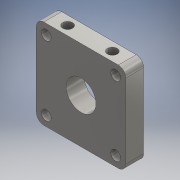
# Autodesk Inventor part: Bearing_Block
Saved by Autodesk Inventor 2016 (Build 200138000, 138)
## iProperties
Created: 2016-04-11
Part Number: Bearing_Block
Material: Steel, Mild
Document SubType Name: Modeling
Designer: agmle
Density: 7.85 g/cm^3
Appearance: Semi-Polished
Author: agmle
Autodesk Inventor part; units mm, degrees
ref_plane "YZ Plane" through (0, 0, 0) normal (1, 0, 0) x (0, 1, 0)
ref_plane "XZ Plane" through (0, 0, 0) normal (0, 1, 0) x (-1, 0, 0)
ref_plane "XY Plane" through (0, 0, 0) normal (0, 0, 1) x (1, 0, 0)
sketch "Sketch1" plane through (0, 0, 0) normal (0, 1, 0) x (-1, 0, 0)
  line L0 (16.6369, 20.0223) -> (-15.1131, 20.0223)
  line L1 (-18.2881, 16.8473) -> (-18.2881, -14.9027)
  line L2 (-15.1131, -18.0777) -> (16.6369, -18.0777)
  line L3 (19.8119, -14.9027) -> (19.8119, 16.8473)
  arc A0 (19.8119, 16.8473) -> (16.6369, 20.0223) centre (16.6369, 16.8473) ccw
  arc A1 (-18.2881, -14.9027) -> (-15.1131, -18.0777) centre (-15.1131, -14.9027) ccw
  arc A2 (16.6369, -18.0777) -> (19.8119, -14.9027) centre (16.6369, -14.9027) ccw
  arc A3 (-15.1131, 20.0223) -> (-18.2881, 16.8473) centre (-15.1131, 16.8473) ccw
  point P0 (0, 0)
  dimension "d0" = 38.1
  dimension "d1" = 3.175
  constraints: 8 end point, 8 point on circle, 8 tangent, 4 centre point, 3 equal radius, 2 parallel, 2 perpendicular, 1 horizontal
  measures "d0" distance between parallel lines of L2 L0
  measures "d1" radius of A0
extrude "Extrusion1" add sketch "Sketch1" along normal blind 7.62
sketch "Sketch2" plane through (0, 7.62, 0) normal (0, 1, 0) x (1, 0, 0)
  line L0 (-19.8119, 14.9027) -> (-19.8119, -16.8473) projected
  line L1 (-16.6369, -20.0223) -> (15.1131, -20.0223) projected
  line L2 (15.1131, 18.0777) -> (-16.6369, 18.0777) projected
  line L3 (18.2881, -16.8473) -> (18.2881, 14.9027) projected
  point P0 (0, 0)
  point P1 (-15.5619, -15.7723)
  point P2 (-15.5619, 13.8277)
  point P3 (14.0381, 13.8277)
  point P4 (14.0381, -15.7723)
  dimension "d4" = 4.25
  dimension "d5" = 4.25
  dimension "d6" = 4.25
  dimension "d7" = 4.25
  dimension "d8" = 4.25
  dimension "d9" = 4.25
  dimension "d10" = 4.25
  dimension "d11" = 4.25
  measures "d4" distance from line of L0 point (-15.562, -15.772)
  measures "d5" distance from line of L1 point (-15.562, -15.772)
  measures "d6" distance from line of L0 point (-15.562, 13.828)
  measures "d7" distance from line of L2 point (-15.562, 13.828)
  measures "d8" distance from line of L2 point (14.038, 13.828)
  measures "d9" distance from line of L3 point (14.038, 13.828)
  measures "d10" distance from line of L3 point (14.038, -15.772)
  measures "d11" distance from line of L1 point (14.038, -15.772)
hole "Hole1" at (-15.5619, 7.62, 15.7723) at (-15.5619, 7.62, -13.8277) at (14.0381, 7.62, -13.8277) at (14.0381, 7.62, 15.7723) direction (0, -1, 0) diameter 4.2 end through all
sketch "Sketch3" plane through (0, 7.62, 0) normal (0, 1, 0) x (1, 0, 0)
  line L0 (-19.8119, 14.9027) -> (-19.8119, -16.8473) construction
  line L1 (-19.8119, -0.9723) -> (18.2881, -0.9723) construction
  line L2 (18.2881, -16.8473) -> (18.2881, 14.9027) construction
  point P0 (0, 0)
  point P1 (-0.7619, -0.9723)
  point P2 (-0.7619, -0.9723)
  constraints: 3 midpoint, 2 end point, 1 coincident
hole "Hole2" at (-0.7619, 7.62, 0.9723) direction (0, -1, 0) diameter 12.7 end through all
sketch "Sketch4" plane through (-16.6369, 0, 20.0223) normal (0, 0, 1) x (1, 0, 0)
  line L0 (31.75, 0) -> (31.75, 7.62) construction
  line L1 (31.75, 3.81) -> (0, 3.81) construction
  line L2 (0, 0) -> (0, 7.62) construction
  line L3 (-3.175, 0) -> (-3.175, 7.62) construction
  line L4 (34.925, 0) -> (34.925, 7.62) construction
  point P0 (16.6369, 0)
  point P1 (6.35, 3.81)
  point P2 (25.4, 3.81)
  dimension "d26" = 9.525
  dimension "d27" = 9.525
  constraints: 2 end point, 2 midpoint, 2 point on line
  measures "d26" distance from line of L3 point (6.35, 3.81)
  measures "d27" distance from line of L4 point (25.4, 3.81)
hole "Hole3" at (-10.2869, 3.81, 20.0223) at (8.7631, 3.81, 20.0223) direction (0, 0, -1) diameter 4.2 depth 7.62 tip angle 118
sketch "Sketch5" plane through (15.1131, 0, -18.0777) normal (0, 0, -1) x (-1, 0, 0)
  line L0 (-3.175, 0) -> (-3.175, 7.62) construction
  line L1 (34.925, 0) -> (34.925, 7.62) construction
  line L2 (31.75, 0) -> (31.75, 7.62) construction
  line L3 (0, 0) -> (0, 7.62) construction
  line L4 (0, 0) -> (0, 7.62) construction
  line L5 (0, 3.81) -> (31.75, 3.81) construction
  line L6 (31.75, 0) -> (31.75, 7.62) construction
  point P0 (15.1131, 0)
  point P1 (6.35, 3.81)
  point P2 (25.4, 3.81)
  dimension "d35" = 9.525
  dimension "d36" = 9.525
  constraints: 2 end point, 2 midpoint, 2 point on line
  measures "d35" distance from line of L1 point (25.4, 3.81)
  measures "d36" distance from line of L0 point (6.35, 3.81)
hole "Hole4" at (8.7631, 3.81, -18.0777) at (-10.2869, 3.81, -18.0777) direction (0, 0, 1) diameter 4.2 depth 7.62 tip angle 118
equation "\"d5\" = d4"
equation "\"d6\" = d4"
equation "\"d7\" = d4"
equation "\"d8\" = d4"
equation "\"d9\" = d4"
equation "\"d10\" = d4"
equation "\"d11\" = d4"
equation "\"d27\" = d26"
equation "\"d35\" = d26"
equation "\"d36\" = d26"
body "Solid1"
